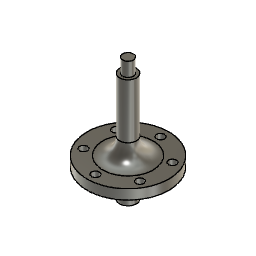
acople_motor_turbina (Autodesk Fusion 360 design; units mm, degrees)
Autodesk Fusion 360 part; units mm, degrees
sketch "Boceto1" plane through (0, 0, 0) normal (0, 0, 1) x (1, 0, 0)
  circle A0 centre (0, 0) radius 29.2
  circle A1 centre (0, 23.3) radius 2.8
  circle A2 centre (-20.1784, 11.65) radius 2.8
  circle A3 centre (-20.1784, -11.65) radius 2.8
  circle A4 centre (0, -23.3) radius 2.8
  circle A5 centre (20.1784, -11.65) radius 2.8
  circle A6 centre (20.1784, 11.65) radius 2.8
  dimension "d1" = 58.4
  dimension "d2" = 5.6
  dimension "d4" = 360
  dimension "d14" = 23.3
  constraint coincident A0.centre origin
  measures "d1" diameter of A0
  measures "d2" diameter of A1
  measures "d14" distance of A0.centre A1.centre
extrude "Extruir1" add sketch "Boceto1" against normal blind 7
sketch "Boceto2" plane through (0, 0, 0) normal (0, 0, 1) x (-1, 0, 0)
  circle A0 centre (0, -23.3) radius 2.8
  circle A1 centre (20.1784, 11.65) radius 2.8
  circle A2 centre (20.1784, -11.65) radius 2.8
  circle A3 centre (0, 23.3) radius 2.8
  circle A4 centre (-20.1784, 11.65) radius 2.8
  circle A5 centre (-20.1784, -11.65) radius 2.8
  circle A6 centre (0, 0) radius 29.2
  circle A7 centre (0, 0) radius 6
  dimension "d7" = 12
  constraint concentric A6 A7
  measures "d7" diameter of A7
extrude "Extruir2" add sketch "Boceto2" along normal blind 51 contours A7
sketch "Boceto3" plane through (0, 0, 51) normal (0, 0, 1) x (-1, 0, 0)
  circle A0 centre (0, 0) radius 6
  circle A1 centre (0, 0) radius 3.85
  dimension "d10" = 7.7
  constraint concentric A0 A1
  measures "d10" diameter of A1
extrude "Extruir3" add sketch "Boceto3" along normal blind 10 contours A1
sketch "Boceto4" plane through (0, 0, 0) normal (0, 0, 1) x (-1, 0, 0)
  circle A0 centre (0, 0) radius 6
  circle A1 centre (0, -23.3) radius 2.8
  circle A2 centre (20.1784, 11.65) radius 2.8
  circle A3 centre (20.1784, -11.65) radius 2.8
  circle A4 centre (0, 23.3) radius 2.8
  circle A5 centre (-20.1784, 11.65) radius 2.8
  circle A6 centre (-20.1784, -11.65) radius 2.8
  circle A7 centre (0, 0) radius 29.2
  circle A8 centre (0, 0) radius 20.3
  dimension "d13" = 40.6
  constraint concentric A0 A8
  measures "d13" diameter of A8
sketch "Boceto5" plane through (0, 0, 0) normal (0, 1, 0) x (1, 0, 0)
fillet "Empalme1" radius 12 1 edges at (5.594, -2.1697, 0)
sketch "Boceto6" plane through (0, 0, -7) normal (0, 0, -1) x (1, 0, 0)
  circle A0 centre (0, -23.3) radius 2.8
  circle A1 centre (-20.1784, -11.65) radius 2.8
  circle A2 centre (-20.1784, 11.65) radius 2.8
  circle A3 centre (0, 23.3) radius 2.8
  circle A4 centre (20.1784, 11.65) radius 2.8
  circle A5 centre (20.1784, -11.65) radius 2.8
  circle A6 centre (0, 0) radius 29.2
  circle A7 centre (0, 0) radius 6
  dimension "d17" = 12
  constraint concentric A6 A7
  measures "d17" diameter of A7
extrude "Extruir4" add sketch "Boceto6" along normal blind 20 contours A7
